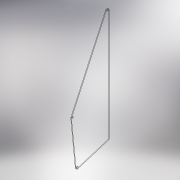
# Autodesk Inventor part: swan_plate
Saved by Autodesk Inventor 2018.2 (Build 222227000, 227)
## iProperties
Created: 2017-12-11
Part Number: swan_plate
Material: 一般
Document SubType Name: Modeling
Designer: kuwano
Density: 1 g/cm^3
Appearance: 既定
Author: kuwano
Autodesk Inventor part; units mm, degrees
ref_plane "YZ Plane" through (0, 0, 0) normal (1, 0, 0) x (0, 1, 0)
ref_plane "XZ Plane" through (0, 0, 0) normal (0, 1, 0) x (-1, 0, 0)
ref_plane "XY Plane" through (0, 0, 0) normal (0, 0, 1) x (1, 0, 0)
sketch "スケッチ1" plane through (0, 0, 0) normal (1, 0, 0) x (0, 1, 0)
  circle A0 centre (0, 0) radius 4
  circle A1 centre (30, -300) radius 4
  circle A2 centre (230, 350) radius 4
  line L0 (248.6746, 396.6269) -> (151.2885, -136.9946)
  line L1 (151.2885, -136.9946) -> (22.8179, -328.6776)
  line L2 (22.8179, -328.6776) -> (-10.3029, 2.5306)
  line L3 (248.6746, 396.6269) -> (-10.3029, 2.5306)
  dimension "d0" = 30
  dimension "d1" = 300
  dimension "d2" = 8
  dimension "d3" = 8
  dimension "d4" = 350
  dimension "d5" = 230
  dimension "d6" = 8
  dimension "d9" = 10
  dimension "d11" = 10
  dimension "d13" = 10
  dimension "d14" = 10
  dimension "d16" = 10
  dimension "d29" = 10
  constraints: 8 end point, 3 centre point, 1 coincident
  measures "d0" horizontal distance of A1.centre point (0, 0)
  measures "d1" vertical distance of point (0, 0) A1.centre
  measures "d2" diameter of A0
  measures "d3" diameter of A1
  measures "d4" vertical distance of point (0, 0) A2.centre
  measures "d5" horizontal distance of point (0, 0) A2.centre
  measures "d6" diameter of A2
  measures "d9" distance from line of A2.centre L0
  measures "d11" distance from line of L2 point (0, 0)
  measures "d13" distance from line of L1 A1.centre
  measures "d14" distance from line of L2 A1.centre
  measures "d16" distance from line of L3 A2.centre
  measures "d29" distance from line of point (0, 0) L3
extrude "押し出し3" add sketch "スケッチ1" along normal mid plane 5
fillet "フィレット3" radius 10 3 edges at (0, 248.6746, 396.6269) (0, 22.8179, -328.6776) (0, -10.3029, 2.5306)
